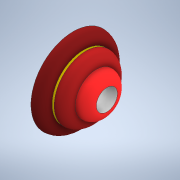
# Autodesk Inventor part: head
Saved by Autodesk Inventor 2021 (Build 250183000, 183)
## iProperties
Created: 2021-07-29
Part Number: head
Material: Generic
Document SubType Name: Modeling
Designer: Shammy Haider
Density: 1 g/cm^3
Appearance: Default
Author: Shammy Haider
Autodesk Inventor part; units mm, degrees
ref_plane "YZ Plane" through (0, 0, 0) normal (1, 0, 0) x (0, 1, 0)
ref_plane "XZ Plane" through (0, 0, 0) normal (0, 1, 0) x (-1, 0, 0)
ref_plane "XY Plane" through (0, 0, 0) normal (0, 0, 1) x (1, 0, 0)
sketch "Sketch1" plane through (0, 0, 0) normal (0, 0, 1) x (1, 0, 0)
  line L0 (0, 0) -> (0, 20)
  line L1 (0, 20) -> (5, 20)
  line L2 (5, 20) -> (5, 15)
  line L3 (5, 15) -> (11, 15)
  line L4 (11, 15) -> (11, 10)
  line L5 (11, 10) -> (16, 10)
  line L6 (16, 10) -> (16, 5)
  line L7 (16, 5) -> (5, 5)
  line L8 (5, 5) -> (5, 0)
  line L9 (5, 0) -> (0, 0)
  dimension "d0" = 20
  dimension "d1" = 5
  dimension "d2" = 15
  dimension "d3" = 6
  dimension "d4" = 10
  dimension "d5" = 5
  dimension "d6" = 5
  dimension "d7" = 5
  constraints: 20 end point, 9 perpendicular, 1 vertical
  measures "d0" distance of L0.start L0.end
  measures "d1" distance between parallel lines of L0 L2
  measures "d2" distance between parallel lines of L9 L3
  measures "d3" distance between parallel lines of L2 L4
  measures "d4" distance between parallel lines of L9 L5
  measures "d5" distance between parallel lines of L6 L4
  measures "d6" distance between parallel lines of L9 L7
  measures "d7" distance between parallel lines of L0 L8
revolve "Revolution1" add sketch "Sketch1" angle 360 about axis through (5, 0, 0) along (-1, 0, 0)
fillet "Fillet1" radius 5 3 edges at (5, -20, 0) (11, -15, 0) (16, -10, 0)
body "Solid1"
